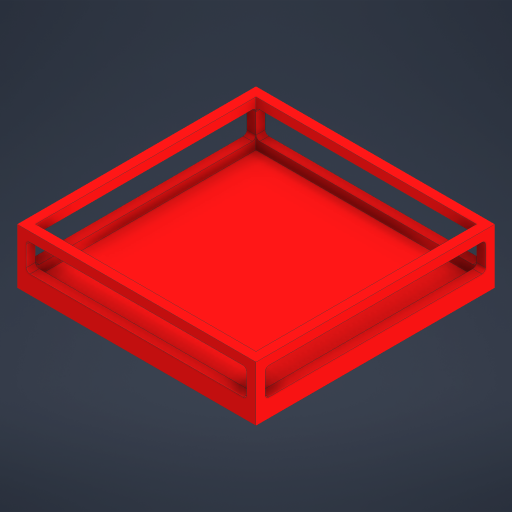
# Autodesk Inventor part: FP V2 Ground Support
Saved by Autodesk Inventor 2023.6 (Build 276521000, 521)
## iProperties
Created: 2026-02-19
Part Number: FP V2 Ground Support
Material: Generic
Document SubType Name: Modeling
Designer: user
Density: 1 g/cm^3
Appearance: Default
Author: user
Autodesk Inventor part; units mm, degrees
ref_plane "YZ Plane" through (0, 0, 0) normal (1, 0, 0) x (0, 1, 0)
ref_plane "XZ Plane" through (0, 0, 0) normal (0, 1, 0) x (-1, 0, 0)
ref_plane "XY Plane" through (0, 0, 0) normal (0, 0, 1) x (1, 0, 0)
sketch "Sketch1" plane through (0, 0, 0) normal (0, 1, 0) x (-1, 0, 0)
  line L0 (65, 65) -> (-65, 65)
  line L1 (-65, 65) -> (-65, -65)
  line L2 (-65, -65) -> (65, -65)
  line L3 (65, -65) -> (65, 65)
  line L4 (65, 65) -> (-65, -65) construction
  line L5 (-65, 65) -> (65, -65) construction
  point P0 (0, 0)
  dimension "d0" = 130
  dimension "d1" = 130
  constraints: 12 end point, 2 midpoint, 2 parallel, 1 horizontal, 1 perpendicular
  measures "d0" distance between parallel lines of L1 L3
  measures "d1" distance between parallel lines of L2 L0
extrude "Extrusion1" add sketch "Sketch1" along normal blind 30
shell "Shell1" thickness 5 removed faces 1 at (21.6667, 30, 21.6667)
sketch "Sketch6" plane through (-65, 0, 65) normal (0, 0, 1) x (1, 0, 0)
  line L0 (5, 25) -> (125, 25)
  line L1 (125, 25) -> (125, 10)
  line L2 (125, 10) -> (5, 10)
  line L3 (5, 10) -> (5, 25)
  line L4 (5, 25) -> (125, 10) construction
  line L5 (125, 25) -> (5, 10) construction
  line L6 (0, 0) -> (130, 0) projected
  line L7 (130, 0) -> (130, 30) projected
  line L8 (0, 30) -> (130, 30) projected
  line L9 (0, 0) -> (0, 30) projected
  line L10 (5, 5) -> (125, 5) projected
  line L11 (5, 5) -> (5, 30) projected
  line L12 (125, 30) -> (5, 30) projected
  line L13 (125, 5) -> (125, 30) projected
  point P0 (65, 0)
  point P1 (65, 17.5)
  point P2 (5, 17.5)
  point P3 (125, 17.5)
  dimension "d24" = 15
  dimension "d25" = 5
  constraints: 12 end point, 6 midpoint, 2 parallel, 1 horizontal, 1 perpendicular
  measures "d24" distance between parallel lines of L2 L0
  measures "d25" distance between parallel lines of L8 L0
sketch "Sketch7" plane through (65, 0, 65) normal (1, 0, 0) x (0, 0, -1)
  line L0 (5, 25) -> (125, 25)
  line L1 (125, 25) -> (125, 10)
  line L2 (125, 10) -> (5, 10)
  line L3 (5, 10) -> (5, 25)
  line L4 (5, 25) -> (125, 10) construction
  line L5 (125, 25) -> (5, 10) construction
  line L6 (0, 0) -> (130, 0) projected
  line L7 (130, 0) -> (130, 30) projected
  line L8 (0, 30) -> (130, 30) projected
  line L9 (0, 0) -> (0, 30) projected
  line L10 (5, 5) -> (5, 30) projected
  line L11 (5, 5) -> (5, 30) projected
  line L12 (125, 5) -> (125, 30) projected
  line L13 (125, 5) -> (125, 30) projected
  point P0 (65, 0)
  point P1 (65, 17.5)
  point P2 (5, 12.5)
  point P3 (125, 17.5)
  dimension "d27" = 15
  dimension "d45" = 5
  dimension "d46" = 120
  constraints: 12 end point, 3 midpoint, 2 parallel, 1 horizontal, 1 perpendicular, 1 point on line
  measures "d27" distance between parallel lines of L2 L0
  measures "d45" distance between parallel lines of L8 L0
  measures "d46" distance between parallel lines of L1 L3
sketch "Sketch8" plane through (-65, 0, -65) normal (-1, 0, 0) x (0, 0, 1)
  line L0 (5, 25) -> (125, 25)
  line L1 (125, 25) -> (125, 10)
  line L2 (125, 10) -> (5, 10)
  line L3 (5, 10) -> (5, 25)
  line L4 (5, 25) -> (125, 10) construction
  line L5 (125, 25) -> (5, 10) construction
  line L6 (125, 5) -> (125, 30) projected
  line L7 (130, 0) -> (130, 30) projected
  line L8 (125, 5) -> (125, 30) projected
  line L9 (130, 0) -> (130, 30) projected
  line L10 (130, 30) -> (0, 30) projected
  line L11 (125, 30) -> (5, 30) projected
  line L12 (5, 5) -> (125, 5) projected
  line L13 (5, 5) -> (5, 30) projected
  line L14 (0, 30) -> (130, 30) projected
  line L15 (0, 0) -> (130, 0) projected
  line L16 (0, 0) -> (0, 30) projected
  line L17 (125, 5) -> (5, 5) projected
  line L18 (5, 30) -> (125, 30) projected
  line L19 (5, 5) -> (5, 30) projected
  line L20 (130, 0) -> (0, 0) projected
  line L21 (0, 0) -> (0, 30) projected
  point P0 (65, 0)
  point P1 (65, 17.5)
  point P2 (5, 12.5)
  point P3 (125, 17.5)
  point P4 (5, 17.5)
  dimension "d30" = 15
  dimension "d47" = 5
  dimension "d48" = 120
  constraints: 12 end point, 4 midpoint, 2 parallel, 1 horizontal, 1 perpendicular, 1 point on line
  measures "d30" distance between parallel lines of L2 L0
  measures "d47" distance between parallel lines of L11 L0
  measures "d48" distance of point (5, 17.5) point (125, 17.5)
sketch "Sketch9" plane through (65, 0, -65) normal (0, 0, -1) x (-1, 0, 0)
  line L0 (5, 25) -> (125, 25)
  line L1 (125, 25) -> (125, 10)
  line L2 (125, 10) -> (5, 10)
  line L3 (5, 10) -> (5, 25)
  line L4 (5, 25) -> (125, 10) construction
  line L5 (125, 25) -> (5, 10) construction
  line L6 (130, 0) -> (130, 30) projected
  line L7 (125, 5) -> (125, 30) projected
  line L8 (130, 0) -> (130, 30) projected
  line L9 (125, 5) -> (125, 30) projected
  line L10 (5, 5) -> (5, 30) projected
  line L11 (125, 5) -> (5, 5) projected
  line L12 (5, 30) -> (125, 30) projected
  line L13 (0, 0) -> (0, 30) projected
  line L14 (130, 0) -> (0, 0) projected
  line L15 (130, 30) -> (0, 30) projected
  line L16 (125, 30) -> (5, 30) projected
  line L17 (5, 5) -> (125, 5) projected
  line L18 (5, 5) -> (5, 30) projected
  line L19 (0, 0) -> (0, 30) projected
  line L20 (0, 30) -> (130, 30) projected
  line L21 (0, 0) -> (130, 0) projected
  point P0 (65, 0)
  point P1 (65, 17.5)
  point P2 (5, 17.5)
  point P3 (125, 17.5)
  dimension "d33" = 15
  dimension "d49" = 5
  constraints: 12 end point, 4 midpoint, 2 parallel, 1 horizontal, 1 perpendicular
  measures "d33" distance between parallel lines of L2 L0
  measures "d49" distance between parallel lines of L15 L0
extrude "Extrusion6" cut sketch "Sketch6" against normal blind 10 contours L0 L1 L2 L3
extrude "Extrusion7" cut sketch "Sketch8" against normal blind 10 contours L0 L1 L2 L3
extrude "Extrusion8" cut sketch "Sketch7" against normal blind 10 contours L0 L1 L2 L3
extrude "Extrusion9" cut sketch "Sketch9" against normal blind 10 contours L0 L1 L2 L3
fillet "Fillet4" radius 2 16 edges at (62.5, 10, 60) (62.5, 25, 60) (62.5, 10, -60) (62.5, 25, -60) (60, 10, -62.5) (-60, 10, -62.5) (-60, 25, -62.5) (60, 25, -62.5) (-62.5, 25, -60) (-62.5, 10, -60) (-62.5, 25, 60) (-62.5, 10, 60) (-60, 25, 62.5) (-60, 10, 62.5) (60, 25, 62.5) (60, 10, 62.5)
body "Solid1"
